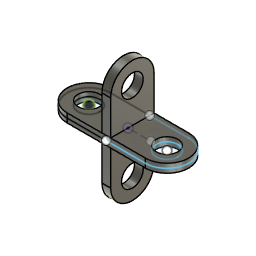
que4 v1 (Autodesk Fusion 360 design; units mm, degrees)
Autodesk Fusion 360 part; units mm, degrees
sketch "Sketch1" plane through (0, 0, 0) normal (0, 0, 1) x (1, 0, 0)
  circle A0 centre (-45, -0.0287) radius 12.5
  line L0 (-45, 24.9713) -> (0, 24.9713)
  line L1 (-45, -25.0287) -> (0, -25.0287)
  circle A1 centre (45, -0.0287) radius 12.5
  line L2 (45, -25.0287) -> (0, -25.0287)
  line L3 (45, 24.9713) -> (0, 24.9713)
  arc A2 (-45, 24.9713) -> (-45, -25.0287) centre (-45, -0.0287) ccw
  arc A3 (45, -25.0287) -> (45, 24.9713) centre (45, -0.0287) ccw
  line L4 (0, 0) -> (26.1946, 0) construction
  dimension "d1" = 25
  dimension "d3" = 50
  constraint concentric A0 A2
  constraint horizontal L0
  constraint tangent L0 A2
  constraint horizontal L1
  constraint tangent L1 A2
  constraint coincident L4.start origin
  constraint parallel L0 L4
  measures "d1" diameter of A0
  measures "d3" diameter of A2
sketch "Sketch2" plane through (0, 0, 0) normal (1, 0, 0) x (0, 1, 0)
  arc A0 (25.0287, 45) -> (-24.9713, 45) centre (0.0287, 45) ccw
  circle A1 centre (0.0287, 45) radius 12.5
  line L0 (-24.9713, -45) -> (-24.9713, -5)
  arc A2 (-24.9713, -45) -> (25.0287, -45) centre (0.0287, -45) ccw
  line L1 (25.0287, -45) -> (25.0287, 0)
  line L2 (25.0287, 45) -> (25.0287, 0)
  circle A3 centre (0.0287, -45) radius 12.5
  line L3 (-24.9713, 45) -> (-24.9713, -5)
  point P0 (0, -5)
  dimension "d4" = 25
  dimension "d6" = 50
  constraint concentric A2 A3
  constraint tangent L0 A2
  constraint tangent A2 L1
  measures "d4" diameter of A3
  measures "d6" diameter of A2
extrude "Extrude1" add sketch "Sketch1" against normal blind 10 makes body 1
extrude "Extrude2" add sketch "Sketch2" along normal blind 10 separate body makes body 2
move_body "Move1" bodies 1 to x (1, 0, 0) y (0, 1, 0) z (0, 0, 1) at (0, 0, 5)
move_body "Move2" bodies 2 to x (1, 0, 0) y (0, 1, 0) z (0, 0, 1) at (-5, 0, 0)
combine "Combine1" operation add target body 1 tool bodies 2
